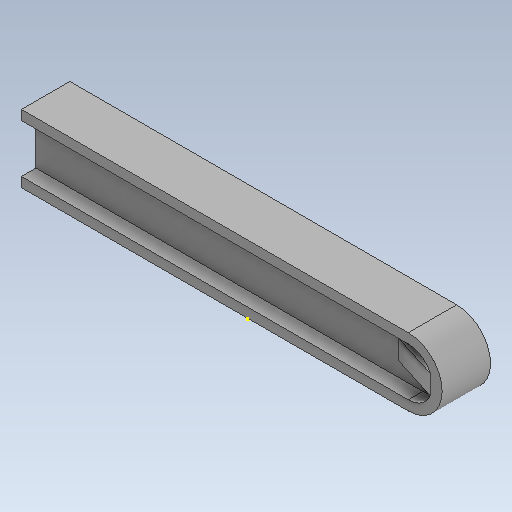
# Autodesk Inventor part: bullet bill
Saved by Autodesk Inventor 2021 (Build 250183000, 183)
## iProperties
Created: 2021-01-30
Part Number: bullet bill
Material: Generic
Document SubType Name: Modeling
Designer: josep
Density: 1 g/cm^3
Appearance: Default
Author: josep
Autodesk Inventor part; units mm, degrees
ref_plane "YZ Plane" through (0, 0, 0) normal (1, 0, 0) x (0, 1, 0)
ref_plane "XZ Plane" through (0, 0, 0) normal (0, 1, 0) x (-1, 0, 0)
ref_plane "XY Plane" through (0, 0, 0) normal (0, 0, 1) x (1, 0, 0)
sketch "Sketch1" plane through (0, 0, 0) normal (1, 0, 0) x (0, 1, 0)
  line L0 (34, 12.5) -> (31, 12.5)
  line L1 (35, 12.5) -> (34, 12.5)
  line L2 (31, 12.5) -> (30, 12.5)
  line L3 (35, -12.5) -> (34, -12.5)
  line L4 (30, -12.5) -> (31, -12.5)
  line L5 (5, -12.5) -> (4, -12.5)
  line L6 (1, -12.5) -> (0, -12.5)
  line L7 (4, 12.5) -> (5, 12.5)
  line L8 (0, 12.5) -> (1, 12.5)
  line L9 (35, 5) -> (0, 5)
  line L10 (0, 5) -> (0, -5)
  line L11 (0, -5) -> (35, -5)
  line L12 (35, -5) -> (35, 5)
  line L13 (0, 12.5) -> (5, 12.5)
  line L14 (5, 12.5) -> (0, 12.5)
  line L15 (0, 12.5) -> (0, 5)
  line L16 (0, 5) -> (5, 5)
  line L17 (5, 5) -> (5, 12.5)
  line L18 (5, -12.5) -> (0, -12.5)
  line L19 (0, -12.5) -> (0, -5)
  line L20 (0, -5) -> (5, -5)
  line L21 (5, -5) -> (5, -12.5)
  line L22 (35, 12.5) -> (30, 12.5)
  line L23 (30, 12.5) -> (30, 5)
  line L24 (30, 5) -> (35, 5)
  line L25 (35, 5) -> (35, 12.5)
  line L26 (35, -12.5) -> (30, -12.5)
  line L27 (30, -12.5) -> (30, -5)
  line L28 (30, -5) -> (35, -5)
  line L29 (35, -5) -> (35, -12.5)
  point P0 (0, 0)
  constraints: 60 end point, 10 parallel, 7 horizontal, 7 point on line, 5 perpendicular
extrude "Extrusion1" add sketch "Sketch1" along normal blind 82.5 and the other way blind 100 contours L1 L25 L9 L23 L2 L0 | L29 L3 L26 L4 L27 L11 | L9 L15 L8 L13 L7 L17 | L21 L5 L18 L6 L19 L11
extrude "Extrusion2" add sketch "Sketch1" along normal mid plane 200 contours L12 L11 L10 L9
sketch "Sketch2" plane through (-100, 0, 5) normal (0, 0, 1) x (1, 0, 0)
  line L0 (200, 0) -> (200, 35) projected
  line L1 (182.5, 35) -> (200, 35) projected
  arc A0 (182.5, 0) -> (182.5, 35) centre (182.5, 17.5) ccw
  line L2 (200, 0) -> (100, 0) projected
  line L3 (182.5, 35) -> (200, 35)
  line L4 (200, 17.5) -> (200, 0)
  line L5 (0, 30) -> (182.5, 30) projected
  arc A1 (182.5, 5) -> (182.5, 30) centre (182.5, 17.5) ccw
  line L6 (182.5, 30) -> (182.5, 35) projected
  line L7 (182.5, 30) -> (182.5, 35)
  line L8 (0, 5) -> (182.5, 5) projected
  line L9 (182.5, 0) -> (182.5, 5) projected
  line L10 (182.5, 5) -> (182.5, 0)
  point P0 (0, 35)
  point P1 (200, 17.5)
  constraints: 9 end point, 5 point on circle, 2 centre point, 2 tangent, 2 vertical, 1 coincident, 1 collinear, 1 perpendicular, 1 point on line
extrude "Extrusion3" cut sketch "Sketch2" against normal blind 20 contours L2 A0 L0 | A0 L1 L0
extrude "Extrusion4" add sketch "Sketch2" along normal blind 7.5 and the other way blind 17.5 contours A0 L9 A1 L6
sketch "Sketch3" plane through (-100, 5, 5) normal (0, 0, 1) x (1, 0, 0)
  arc A0 (182.5, 0) -> (182.5, 25) centre (182.5, 12.5) ccw projected
  line L0 (195, 12.5) -> (195, 17.5)
  line L1 (195, 12.5) -> (195, 7.5)
  line L2 (195, 17.5) -> (170, 17.5)
  line L3 (170, 17.5) -> (170, 7.5)
  line L4 (170, 7.5) -> (195, 7.5)
  point P0 (100, -5)
  point P1 (193.9564, 7.5)
  point P2 (193.9564, 17.5)
  constraints: 10 end point, 2 perpendicular, 1 horizontal, 1 point on circle, 1 point on line, 1 tangent, 1 vertical
extrude "Extrusion5" add sketch "Sketch3" along normal blind 7.5 and the other way blind 17.5 contours L4 L3 L2 A0
sketch "Sketch4" plane through (70, 22.5, 5) normal (0, 1, 0) x (1, 0, 0)
  line L0 (23.9564, -7.5) -> (0, -7.5) projected
  line L1 (0, 0) -> (23.9564, -7.5)
  line L2 (23.9564, -7.5) -> (0, -7.5)
  line L3 (-170, 17.5) -> (12.5, 17.5) projected
  line L4 (0, -7.5) -> (0, 0)
  point P0 (-70, 5)
  constraints: 6 end point, 1 parallel, 1 perpendicular
extrude "Extrusion6" cut sketch "Sketch4" against normal blind 10
sketch "Sketch5" plane through (70, 22.5, -5) normal (0, 1, 0) x (1, 0, 0)
  line L0 (23.9564, 7.5) -> (23.9564, 0) projected
  line L1 (23.9564, 7.5) -> (0, 0)
  line L2 (0, 7.5) -> (0, 0) projected
  line L3 (0, 0) -> (0, 7.5)
  line L4 (0, 7.5) -> (23.9564, 7.5) projected
  line L5 (0, 7.5) -> (23.9564, 7.5)
  point P0 (-70, -5)
  constraints: 6 end point, 1 perpendicular, 1 vertical
extrude "Extrusion7" cut sketch "Sketch5" against normal blind 10
sketch "Sketch6" plane through (-100, 0, 0) normal (-1, 0, 0) x (0, 0, 1)
  line L0 (-12.5, 35) -> (12.5, 35) projected
  line L1 (-12.5, 35) -> (12.5, 35)
  line L2 (12.5, 30) -> (5, 30) projected
  line L3 (12.5, 35) -> (12.5, 30)
  line L4 (12.5, 30) -> (5, 30)
  line L5 (5, 5) -> (5, 12.5) projected
  line L6 (5, 30) -> (5, 5)
  line L7 (5, 5) -> (12.5, 5)
  line L8 (12.5, 0) -> (12.5, 35) projected
  line L9 (12.5, 5) -> (12.5, 0)
  line L10 (12.5, 0) -> (-12.5, 0) projected
  line L11 (12.5, 0) -> (-12.5, 0)
  line L12 (-12.5, 5) -> (-5, 5) projected
  line L13 (-12.5, 0) -> (-12.5, 5)
  line L14 (-12.5, 5) -> (-5, 5)
  line L15 (-5, 5) -> (-5, 30)
  line L16 (-5, 30) -> (-12.5, 30)
  line L17 (-12.5, 35) -> (-12.5, 0) projected
  line L18 (-12.5, 30) -> (-12.5, 35)
  point P0 (0, 0)
  constraints: 24 end point, 8 perpendicular, 3 vertical, 2 point on line, 1 horizontal
extrude "Extrusion8" add sketch "Sketch6" along normal blind 17.25 contours L0 L3 L2 L6 L5 L7 L8 L10 L13 L12 L15 L16 L17
sketch "Sketch7" plane through (82.5, 17.5, 12.5) normal (0, 0, 1) x (1, 0, 0)
  point P0 (-82.5, -17.5)
sketch "Sketch8" plane through (-117.25, 0, 0) normal (-1, 0, 0) x (0, 0, 1)
  point P0 (0, 0)
body "Solid1"
